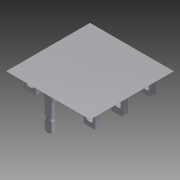
# Autodesk Inventor part: tlD-pins
Saved by Autodesk Inventor 2011 SP1 (Build 150282100, 282)
## iProperties
Created: 2013-12-24
Part Number: tlD-pins
Catalog Web Link: www.cadenas.de
Description: TL Series - Fully Illuminated Toggles - pins-
Vendor: NKKSWITCHES
Document SubType Name: Modeling
Designer: PARTuser1
Manufacturer: NKKSWITCHES
Density: 1 g/cm^3
Category: PARTsolutions
Company: NKKSWITCHES
Title: tlD-pins
Author: Cadenas PARTsolutions
PSOL_IDENT_0: {$CADENAS_DATA\23d-libs\nkkswitches\toggle\tl\parts\tl_pins.prj},198 {VTYP=3D},{NB=tlD-pins},{LINA=t
PSOL_IDENT_1: lD-pins},{NN=TL Series - Fully Illuminated Toggles - pins},{DATE=08.04.2009 12:11:38},{GEOMDATE=26.0
PSOL_IDENT_2: 3.2009 00:00:00},{VERSION=},{LINEID=10},{LINESUBID=-1},{WBVAR=TL}  {NB=tlD-pins},{LINA=tlD-pins},{KT
PSOL_IDENT_3: =DUMMY},{SRS=TL},{PN=tlD-pins},{TL=D},{TCR=W01},{COLOR=SILVER},{COLORALG=0.75,0.75,0.75,0.00}
CNS_NN: TL Series - Fully Illuminated Toggles - pins
CNS_NB: tlD-pins
CNS_NBSYN: $PN.
CNS_LINA: tlD-pins
CNS_SRS: TL
CNS_PN: tlD-pins
CNS_TL: D - .689œ (17.5 mm) (combines with silver contacts only)
CNS_TCR: W01
CNS_COLOR: SILVER
CNS_COLORALG: 0.75,0.75,0.75,0.00
SUPPLIER: NKKSWITCHES
ARTICLENO: tlD-pins
BOMINFO: tlD-pins
CREATOR: CADENAS GmbH
Autodesk Inventor part; units mm, degrees
sketch "Sketch_1" plane through (0, 0, 0) normal (0, 1, 0) x (-1, 0, 0)
  line L0 (7.0485, -7.0485) -> (7.0485, 7.0485)
  line L1 (7.0485, 7.0485) -> (-7.0485, 7.0485)
  line L2 (-7.0485, 7.0485) -> (-7.0485, -7.0485)
  line L3 (-7.0485, -7.0485) -> (7.0485, -7.0485)
  constraints: 8 end point
extrude "Extrusion1" add sketch "Sketch_1" along normal blind 0.0254
sketch "Sketch_3" plane through (0, 0, 7.0485) normal (0, 0, 1) x (1, 0, 0)
  line L0 (-0.7112, 0.0254) -> (-0.7112, -0.7366)
  line L1 (-0.7112, -0.7366) -> (-0.5842, -0.7366)
  line L2 (-0.5842, -0.7366) -> (-0.5842, -3.048)
  line L3 (-0.5842, -3.048) -> (-0.4318, -3.048)
  line L4 (-0.4318, -3.048) -> (-0.4318, -3.556)
  line L5 (-0.4318, -3.556) -> (-0.5842, -3.556)
  line L6 (-0.5842, -3.556) -> (-0.5842, -5.08)
  arc A0 (-0.5842, -5.08) -> (0.5842, -5.08) centre (0, -4.772) ccw
  line L7 (0.5842, -5.08) -> (0.5842, -3.556)
  line L8 (0.5842, -3.556) -> (0.4318, -3.556)
  line L9 (0.4318, -3.556) -> (0.4318, -3.048)
  line L10 (0.4318, -3.048) -> (0.5842, -3.048)
  line L11 (0.5842, -3.048) -> (0.5842, -0.7366)
  line L12 (0.5842, -0.7366) -> (0.7112, -0.7366)
  line L13 (0.7112, -0.7366) -> (0.7112, 0.0254)
  line L14 (0.7112, 0.0254) -> (-0.7112, 0.0254)
  constraints: 30 end point, 2 point on circle, 1 centre point
extrude "Extrusion2" add sketch "Sketch_3" against normal blind 0.6096
sketch "Sketch_5" plane through (0, 0, 0) normal (0, 0, 1) x (1, 0, 0)
  line L0 (4.0005, 0.0254) -> (4.0005, -3.2512)
  arc A0 (4.0005, -3.2512) -> (4.2545, -3.5052) centre (4.2545, -3.2512) ccw
  line L1 (4.2545, -3.5052) -> (5.7531, -3.5052)
  arc A1 (5.7531, -3.5052) -> (6.0071, -3.2512) centre (5.7531, -3.2512) ccw
  line L2 (6.0071, -3.2512) -> (6.0071, 0.0254)
  line L3 (6.0071, 0.0254) -> (4.0005, 0.0254)
  arc A2 (4.4577, -2.3876) -> (5.5499, -2.3876) centre (5.0038, -0.8728) ccw
  line L4 (5.5499, -2.3876) -> (5.5499, -0.5842)
  arc A3 (5.5499, -0.5842) -> (4.4577, -0.5842) centre (5.0038, -1.9147) ccw
  line L5 (4.4577, -0.5842) -> (4.4577, -2.3876)
  constraints: 12 end point, 8 point on circle, 4 centre point
extrude "Extrusion3" add sketch "Sketch_5" along normal mid plane 0.7874
sketch "Sketch_6" plane through (0, 0, 0) normal (0, 0, 1) x (1, 0, 0)
  line L0 (-6.0071, 0.0254) -> (-6.0071, -3.2512)
  arc A0 (-6.0071, -3.2512) -> (-5.7531, -3.5052) centre (-5.7531, -3.2512) ccw
  line L1 (-5.7531, -3.5052) -> (-4.2545, -3.5052)
  arc A1 (-4.2545, -3.5052) -> (-4.0005, -3.2512) centre (-4.2545, -3.2512) ccw
  line L2 (-4.0005, -3.2512) -> (-4.0005, 0.0254)
  line L3 (-4.0005, 0.0254) -> (-6.0071, 0.0254)
  line L4 (-5.5499, -0.5842) -> (-5.5499, -2.3876)
  arc A2 (-5.5499, -2.3876) -> (-4.4577, -2.3876) centre (-5.0038, -0.8728) ccw
  line L5 (-4.4577, -2.3876) -> (-4.4577, -0.5842)
  arc A3 (-4.4577, -0.5842) -> (-5.5499, -0.5842) centre (-5.0038, -1.9147) ccw
  constraints: 12 end point, 8 point on circle, 4 centre point
extrude "Extrusion4" add sketch "Sketch_6" along normal mid plane 0.7874
sketch "Sketch_7" plane through (0, 0, -4.699) normal (0, 0, 1) x (1, 0, 0)
  line L0 (4.0005, 0.0254) -> (4.0005, -2.7432)
  arc A0 (4.0005, -2.7432) -> (4.2545, -2.9972) centre (4.2545, -2.7432) ccw
  line L1 (4.2545, -2.9972) -> (5.7531, -2.9972)
  arc A1 (5.7531, -2.9972) -> (6.0071, -2.7432) centre (5.7531, -2.7432) ccw
  line L2 (6.0071, -2.7432) -> (6.0071, 0.0254)
  line L3 (6.0071, 0.0254) -> (4.0005, 0.0254)
  arc A2 (4.4577, -2.1336) -> (5.5499, -2.1336) centre (5.0038, -0.6188) ccw
  line L4 (5.5499, -2.1336) -> (5.5499, -0.3302)
  arc A3 (5.5499, -0.3302) -> (4.4577, -0.3302) centre (5.0038, -1.6607) ccw
  line L5 (4.4577, -0.3302) -> (4.4577, -2.1336)
  constraints: 12 end point, 8 point on circle, 4 centre point
extrude "Extrusion5" add sketch "Sketch_7" along normal mid plane 0.7874
sketch "Sketch_8" plane through (0, 0, -4.699) normal (0, 0, 1) x (1, 0, 0)
  line L0 (-6.0071, 0.0254) -> (-6.0071, -2.7432)
  arc A0 (-6.0071, -2.7432) -> (-5.7531, -2.9972) centre (-5.7531, -2.7432) ccw
  line L1 (-5.7531, -2.9972) -> (-4.2545, -2.9972)
  arc A1 (-4.2545, -2.9972) -> (-4.0005, -2.7432) centre (-4.2545, -2.7432) ccw
  line L2 (-4.0005, -2.7432) -> (-4.0005, 0.0254)
  line L3 (-4.0005, 0.0254) -> (-6.0071, 0.0254)
  line L4 (-5.5499, -0.3302) -> (-5.5499, -2.1336)
  arc A2 (-5.5499, -2.1336) -> (-4.4577, -2.1336) centre (-5.0038, -0.6188) ccw
  line L5 (-4.4577, -2.1336) -> (-4.4577, -0.3302)
  arc A3 (-4.4577, -0.3302) -> (-5.5499, -0.3302) centre (-5.0038, -1.6607) ccw
  constraints: 12 end point, 8 point on circle, 4 centre point
extrude "Extrusion6" add sketch "Sketch_8" along normal mid plane 0.7874
sketch "Sketch_9" plane through (0, 0, 4.699) normal (0, 0, 1) x (1, 0, 0)
  line L0 (4.0005, 0.0254) -> (4.0005, -2.7432)
  arc A0 (4.0005, -2.7432) -> (4.2545, -2.9972) centre (4.2545, -2.7432) ccw
  line L1 (4.2545, -2.9972) -> (5.7531, -2.9972)
  arc A1 (5.7531, -2.9972) -> (6.0071, -2.7432) centre (5.7531, -2.7432) ccw
  line L2 (6.0071, -2.7432) -> (6.0071, 0.0254)
  line L3 (6.0071, 0.0254) -> (4.0005, 0.0254)
  arc A2 (4.4577, -2.1336) -> (5.5499, -2.1336) centre (5.0038, -0.6188) ccw
  line L4 (5.5499, -2.1336) -> (5.5499, -0.3302)
  arc A3 (5.5499, -0.3302) -> (4.4577, -0.3302) centre (5.0038, -1.6607) ccw
  line L5 (4.4577, -0.3302) -> (4.4577, -2.1336)
  constraints: 12 end point, 8 point on circle, 4 centre point
extrude "Extrusion7" add sketch "Sketch_9" along normal mid plane 0.7874
sketch "Sketch_10" plane through (0, 0, 4.699) normal (0, 0, 1) x (1, 0, 0)
  line L0 (-6.0071, 0.0254) -> (-6.0071, -2.7432)
  arc A0 (-6.0071, -2.7432) -> (-5.7531, -2.9972) centre (-5.7531, -2.7432) ccw
  line L1 (-5.7531, -2.9972) -> (-4.2545, -2.9972)
  arc A1 (-4.2545, -2.9972) -> (-4.0005, -2.7432) centre (-4.2545, -2.7432) ccw
  line L2 (-4.0005, -2.7432) -> (-4.0005, 0.0254)
  line L3 (-4.0005, 0.0254) -> (-6.0071, 0.0254)
  line L4 (-5.5499, -0.3302) -> (-5.5499, -2.1336)
  arc A2 (-5.5499, -2.1336) -> (-4.4577, -2.1336) centre (-5.0038, -0.6188) ccw
  line L5 (-4.4577, -2.1336) -> (-4.4577, -0.3302)
  arc A3 (-4.4577, -0.3302) -> (-5.5499, -0.3302) centre (-5.0038, -1.6607) ccw
  constraints: 12 end point, 8 point on circle, 4 centre point
extrude "Extrusion8" add sketch "Sketch_10" along normal mid plane 0.7874
sketch "Sketch_4" plane through (0, 0, -7.0485) normal (0, 0, 1) x (1, 0, 0)
  line L0 (-0.7112, 0.0254) -> (-0.7112, -0.7366)
  line L1 (-0.7112, -0.7366) -> (-0.5842, -0.7366)
  line L2 (-0.5842, -0.7366) -> (-0.5842, -3.048)
  line L3 (-0.5842, -3.048) -> (-0.4318, -3.048)
  line L4 (-0.4318, -3.048) -> (-0.4318, -3.556)
  line L5 (-0.4318, -3.556) -> (-0.5842, -3.556)
  line L6 (-0.5842, -3.556) -> (-0.5842, -5.08)
  arc A0 (-0.5842, -5.08) -> (0.5842, -5.08) centre (0, -4.772) ccw
  line L7 (0.5842, -5.08) -> (0.5842, -3.556)
  line L8 (0.5842, -3.556) -> (0.4318, -3.556)
  line L9 (0.4318, -3.556) -> (0.4318, -3.048)
  line L10 (0.4318, -3.048) -> (0.5842, -3.048)
  line L11 (0.5842, -3.048) -> (0.5842, -0.7366)
  line L12 (0.5842, -0.7366) -> (0.7112, -0.7366)
  line L13 (0.7112, -0.7366) -> (0.7112, 0.0254)
  line L14 (0.7112, 0.0254) -> (-0.7112, 0.0254)
  constraints: 30 end point, 2 point on circle, 1 centre point
extrude "Extrusion9" add sketch "Sketch_4" along normal blind 0.6096
ref_plane "pins_to_body_XY" through (0, 0, 0) normal (0, -1, 0) x (1, 0, 0)
ref_plane "pins_to_body_YZ" through (0, 0, 0) normal (1, 0, 0) x (0, 0, 1)
ref_plane "pins_to_body_ZX" through (0, 0, 0) normal (0, 0, 1) x (0, -1, 0)
body "Solid1"
